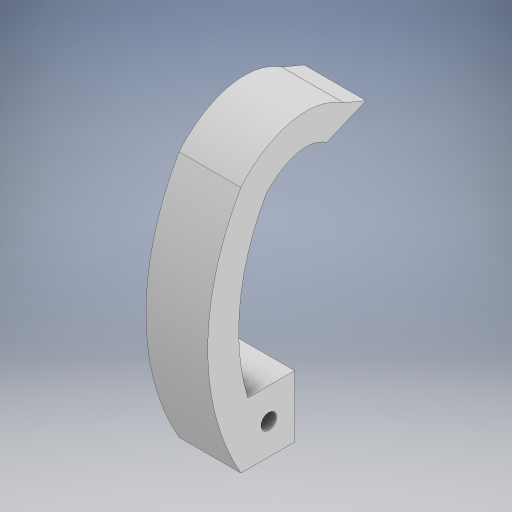
# Autodesk Inventor part: hook4
Saved by Autodesk Inventor 2024.2 (Build 282272000, 272)
## iProperties
Created: 2024-03-12
Part Number: hook4
Material: Generic
Document SubType Name: Modeling
Designer: rohan
Density: 1 g/cm^3
Appearance: Default
Author: rohan
Autodesk Inventor part; units mm, degrees
ref_plane "YZ Plane" through (0, 0, 0) normal (1, 0, 0) x (0, 1, 0)
ref_plane "XZ Plane" through (0, 0, 0) normal (0, 1, 0) x (-1, 0, 0)
ref_plane "XY Plane" through (0, 0, 0) normal (0, 0, 1) x (1, 0, 0)
sketch "Sketch1" plane through (0, 0, 0) normal (1, 0, 0) x (0, 1, 0)
  circle A0 centre (-5090.5276, 4554.0131) radius 3.175
  line L0 (-5103.2276, 4565.4382) -> (-5077.8276, 4565.4382)
  line L1 (-5103.2276, 4565.4382) -> (-5103.2276, 4543.3576)
  line L2 (-5103.2276, 4543.3576) -> (-5077.8276, 4543.3576)
  line L3 (-5077.8276, 4543.3576) -> (-5077.8276, 4565.4382)
  arc A1 (-5001.6276, 4565.4382) -> (-5103.2276, 4565.4382) centre (-5052.4276, 4477.45) ccw
  line L4 (-5001.6276, 4565.4382) -> (-5001.6276, 4565.4382) construction
  line L5 (-5001.6276, 4565.4382) -> (-4980.3953, 4549.1013) construction
  line L6 (-4980.3953, 4549.1013) -> (-4987.2176, 4531.3606) construction
  line L7 (-4987.2176, 4531.3606) -> (-4992.573, 4523.2204) construction
  spline S0 degree 4 poles (-5001.6276, 4565.4382) (-5001.6064, 4565.4219) (-4980.3953, 4549.1013) (-4987.2176, 4531.3606) (-4992.573, 4523.2204) knots 1 1 1 1 1 2 2 2 2 2
  arc A2 (-5008.9368, 4554.9856) -> (-5096.8776, 4554.4397) centre (-5052.4276, 4477.45) ccw
  line L8 (-5003.1828, 4530.2006) -> (-4996.4289, 4514.0091)
  line L9 (-4996.4289, 4514.0091) -> (-4992.573, 4523.2204)
  spline S1 degree 5 poles (-5008.9364, 4554.986) (-5008.9276, 4554.9781) (-5008.9188, 4554.9701) (-5008.9101, 4554.9622) (-5008.8623, 4554.9187) (-5008.8147, 4554.8751) (-5008.7759, 4554.8393) (-5008.6939, 4554.7632) (-5008.6123, 4554.6866) (-5008.5693, 4554.646) (-5008.4793, 4554.5605) (-5008.3898, 4554.4744) (-5008.3431, 4554.4291) (-5008.2459, 4554.3345) (-5008.1494, 4554.2392) (-5008.0993, 4554.1895) (-5007.9958, 4554.0861) (-5007.8931, 4553.9822) (-5007.8402, 4553.9282) (-5007.7315, 4553.8167) (-5007.6235, 4553.7045) (-5007.5682, 4553.6466) (-5007.455, 4553.5274) (-5007.3427, 4553.4074) (-5007.2853, 4553.3457) (-5007.1684, 4553.2191) (-5007.0525, 4553.0916) (-5006.9934, 4553.0263) (-5006.8737, 4552.8928) (-5006.7549, 4552.7585) (-5006.6947, 4552.6898) (-5006.5728, 4552.5499) (-5006.452, 4552.4091) (-5006.3909, 4552.3373) (-5006.2675, 4552.1914) (-5006.1454, 4552.0445) (-5006.0837, 4551.9698) (-5005.9596, 4551.8182) (-5005.8368, 4551.6657) (-5005.7749, 4551.5883) (-5005.6508, 4551.4316) (-5005.5279, 4551.2739) (-5005.4662, 4551.1941) (-5005.3425, 4551.0326) (-5005.2203, 4550.8702) (-5005.159, 4550.7881) (-5005.0364, 4550.6224) (-5004.9153, 4550.4556) (-5004.8547, 4550.3715) (-5004.7338, 4550.2019) (-5004.6143, 4550.0312) (-5004.5547, 4549.9452) (-5004.4359, 4549.7722) (-5004.3187, 4549.5981) (-5004.2603, 4549.5105) (-5004.1441, 4549.3345) (-5004.0296, 4549.1573) (-5003.9726, 4549.0683) (-5003.8594, 4548.8896) (-5003.748, 4548.7099) (-5003.6927, 4548.6197) (-5003.5829, 4548.4388) (-5003.475, 4548.2568) (-5003.4215, 4548.1656) (-5003.3155, 4547.9829) (-5003.2114, 4547.7991) (-5003.1599, 4547.707) (-5003.0581, 4547.5229) (-5002.9582, 4547.3377) (-5002.9088, 4547.245) (-5002.8113, 4547.0598) (-5002.7159, 4546.8735) (-5002.6688, 4546.7804) (-5002.576, 4546.5945) (-5002.4852, 4546.4075) (-5002.4405, 4546.3142) (-5002.3525, 4546.1278) (-5002.2666, 4545.9405) (-5002.2244, 4545.847) (-5002.1414, 4545.6606) (-5002.0606, 4545.4733) (-5002.0209, 4545.3799) (-5001.9431, 4545.1937) (-5001.8675, 4545.0067) (-5001.8305, 4544.9135) (-5001.7579, 4544.7278) (-5001.6876, 4544.5413) (-5001.6532, 4544.4484) (-5001.5861, 4544.2636) (-5001.5211, 4544.0779) (-5001.4894, 4543.9855) (-5001.4276, 4543.8016) (-5001.3681, 4543.617) (-5001.3391, 4543.5252) (-5001.2827, 4543.3425) (-5001.2286, 4543.1592) (-5001.2024, 4543.068) (-5001.1514, 4542.8867) (-5001.1027, 4542.7048) (-5001.0791, 4542.6144) (-5001.0335, 4542.4347) (-5000.9902, 4542.2544) (-5000.9693, 4542.1648) (-5000.929, 4541.9867) (-5000.891, 4541.8082) (-5000.8728, 4541.7195) (-5000.8378, 4541.5432) (-5000.8051, 4541.3665) (-5000.7894, 4541.2787) (-5000.7596, 4541.1042) (-5000.7321, 4540.9294) (-5000.719, 4540.8425) (-5000.6942, 4540.67) (-5000.6718, 4540.4971) (-5000.6613, 4540.4113) (-5000.6415, 4540.2406) (-5000.6241, 4540.0698) (-5000.6161, 4539.9849) (-5000.6012, 4539.8162) (-5000.5887, 4539.6473) (-5000.583, 4539.5633) (-5000.573, 4539.3965) (-5000.5653, 4539.2296) (-5000.562, 4539.1467) (-5000.5566, 4538.9818) (-5000.5536, 4538.8168) (-5000.5526, 4538.7348) (-5000.5519, 4538.5718) (-5000.5534, 4538.4087) (-5000.5547, 4538.3277) (-5000.5585, 4538.1664) (-5000.5645, 4538.0052) (-5000.568, 4537.925) (-5000.5762, 4537.7655) (-5000.5866, 4537.6062) (-5000.5923, 4537.5269) (-5000.6048, 4537.3691) (-5000.6195, 4537.2115) (-5000.6273, 4537.1331) (-5000.6441, 4536.977) (-5000.6629, 4536.8211) (-5000.6729, 4536.7436) (-5000.6937, 4536.5891) (-5000.7167, 4536.4349) (-5000.7287, 4536.3582) (-5000.7536, 4536.2054) (-5000.7806, 4536.0529) (-5000.7945, 4535.977) (-5000.8234, 4535.8257) (-5000.8543, 4535.6749) (-5000.8703, 4535.5998) (-5000.903, 4535.4502) (-5000.9377, 4535.3011) (-5000.9556, 4535.2268) (-5000.9921, 4535.0789) (-5001.0305, 4534.9315) (-5001.0502, 4534.8581) (-5001.0904, 4534.7119) (-5001.1324, 4534.5663) (-5001.1538, 4534.4937) (-5001.1975, 4534.3493) (-5001.2431, 4534.2055) (-5001.2662, 4534.1339) (-5001.3133, 4533.9914) (-5001.3622, 4533.8496) (-5001.387, 4533.779) (-5001.4373, 4533.6385) (-5001.4893, 4533.4986) (-5001.5157, 4533.4291) (-5001.5691, 4533.2908) (-5001.6241, 4533.1532) (-5001.6519, 4533.0847) (-5001.7081, 4532.9488) (-5001.7659, 4532.8135) (-5001.7951, 4532.7462) (-5001.854, 4532.6128) (-5001.9143, 4532.48) (-5001.9448, 4532.414) (-5002.006, 4532.2833) (-5002.0687, 4532.1532) (-5002.1002, 4532.0887) (-5002.1635, 4531.9608) (-5002.2282, 4531.8336) (-5002.2607, 4531.7706) (-5002.3259, 4531.6459) (-5002.3923, 4531.5218) (-5002.4257, 4531.4604) (-5002.4923, 4531.339) (-5002.5602, 4531.2182) (-5002.5941, 4531.1585) (-5002.6619, 4531.0406) (-5002.7309, 4530.9234) (-5002.7653, 4530.8655) (-5002.834, 4530.7514) (-5002.9036, 4530.6379) (-5002.9384, 4530.5819) (-5003.0075, 4530.4717) (-5003.0776, 4530.362) (-5003.1124, 4530.3081) (-5003.1475, 4530.2542) (-5003.1828, 4530.2006) knots 0 0 0 0 0 0 0.002126 0.002126 0.002126 0.011602 0.011602 0.011602 0.022223 0.022223 0.022223 0.033906 0.033906 0.033906 0.046588 0.046588 0.046588 0.060164 0.060164 0.060164 0.074554 0.074554 0.074554 0.08969 0.08969 0.08969 0.1055 0.1055 0.1055 0.121902 0.121902 0.121902 0.138829 0.138829 0.138829 0.156222 0.156222 0.156222 0.174012 0.174012 0.174012 0.192134 0.192134 0.192134 0.210533 0.210533 0.210533 0.229157 0.229157 0.229157 0.247947 0.247947 0.247947 0.266856 0.266856 0.266856 0.285836 0.285836 0.285836 0.304844 0.304844 0.304844 0.323838 0.323838 0.323838 0.342782 0.342782 0.342782 0.361638 0.361638 0.361638 0.380376 0.380376 0.380376 0.398968 0.398968 0.398968 0.41739 0.41739 0.41739 0.435615 0.435615 0.435615 0.453628 0.453628 0.453628 0.471416 0.471416 0.471416 0.488961 0.488961 0.488961 0.506256 0.506256 0.506256 0.523296 0.523296 0.523296 0.54008 0.54008 0.54008 0.556602 0.556602 0.556602 0.572868 0.572868 0.572868 0.588884 0.588884 0.588884 0.604657 0.604657 0.604657 0.620193 0.620193 0.620193 0.635508 0.635508 0.635508 0.650614 0.650614 0.650614 0.665522 0.665522 0.665522 0.680248 0.680248 0.680248 0.69481 0.69481 0.69481 0.709221 0.709221 0.709221 0.723495 0.723495 0.723495 0.737649 0.737649 0.737649 0.751695 0.751695 0.751695 0.765645 0.765645 0.765645 0.779509 0.779509 0.779509 0.793297 0.793297 0.793297 0.807013 0.807013 0.807013 0.820662 0.820662 0.820662 0.834244 0.834244 0.834244 0.847758 0.847758 0.847758 0.861199 0.861199 0.861199 0.874557 0.874557 0.874557 0.887824 0.887824 0.887824 0.900986 0.900986 0.900986 0.914025 0.914025 0.914025 0.926921 0.926921 0.926921 0.939655 0.939655 0.939655 0.952202 0.952202 0.952202 0.964536 0.964536 0.964536 0.976629 0.976629 0.976629 0.988459 0.988459 0.988459 1 1 1 1 1 1
  point P0 (0, 0)
  point P1 (-5077.8276, 4562.6442)
  dimension "d0" = 101.6
  dimension "d1" = 101.6
  dimension "d2" = 12.7
  constraints: 12 end point, 6 point on circle, 3 centre point, 2 perpendicular, 1 concentric, 1 tangent, 1 vertical, 6 other
  measures "d0" distance of L0.start L4.start
  measures "d1" radius of A1
  measures "d2" radial gap between concentric circles of A1 A2
extrude "Extrusion1" add sketch "Sketch1" along normal blind 25.4
body "Solid1"
